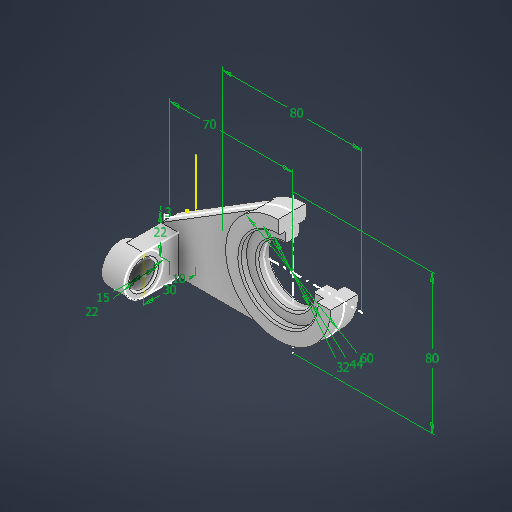
# Autodesk Inventor part: Day02_Task02
Saved by Autodesk Inventor 2026.3 (Build 303398000, 398)
## iProperties
Created: 2026-08-05
Part Number: Day02_Task02
Material: 일반
Document SubType Name: Modeling
Designer: hojin
Density: 1 g/cm^3
Appearance: 기본값
Author: hojin
Autodesk Inventor part; units mm, degrees
ref_plane "YZ Plane" through (0, 0, 0) normal (1, 0, 0) x (0, 1, 0)
ref_plane "XZ Plane" through (0, 0, 0) normal (0, 1, 0) x (-1, 0, 0)
ref_plane "XY Plane" through (0, 0, 0) normal (0, 0, 1) x (1, 0, 0)
sketch "스케치1" plane through (0, 0, 0) normal (0, 1, 0) x (-1, 0, 0)
  point P0 (0, 0)
sketch "스케치2" plane through (0, 0, 0) normal (0, 0, 1) x (1, 0, 0)
  arc A0 (0, 16) -> (16, 0) centre (0, 0) ccw
  arc A1 (0, 22) -> (22, 0) centre (0, 0) ccw
  arc A2 (0, 30) -> (30, 0) centre (0, 0) ccw
  line L0 (-70, -8) -> (-60, -8)
  line L1 (-60, -8) -> (-60, -30)
  line L2 (-60, -30) -> (-70, -30)
  line L3 (-70, -30) -> (-70, -8)
  line L4 (-70, -8) -> (-15.7735, 25.5185)
  line L5 (-70, -30) -> (0, -30)
  line L6 (-73, -8) -> (-70, -8)
  line L7 (-73, -8) -> (-73, -30)
  line L8 (-67, -30) -> (-73, -30)
  line L9 (0, 40) -> (0, -40)
  line L10 (-40, 0) -> (40, 0)
  point P0 (-71.5, -8)
  dimension "d0" = 32
  dimension "d1" = 44
  dimension "d2" = 60
  dimension "d4" = 22
  dimension "d5" = 70
  dimension "d7" = 10
  dimension "d8" = 3
  dimension "d13" = 80
  dimension "d14" = 80
  constraints: 22 end point, 8 point on circle, 6 point on line, 5 coincident, 4 midpoint, 3 centre point, 3 horizontal, 2 parallel, 2 perpendicular, 2 tangent, 2 vertical, 1 collinear
  measures "d0" diameter of A0
  measures "d1" diameter of A1
  measures "d2" diameter of A2
  measures "d4" distance of L0.start L2.end
  measures "d5" horizontal distance of L0.start point (0, 0)
  measures "d7" distance of L1.end L2.end
  measures "d8" distance of L6.start L0.start
  measures "d13" distance of L9.start L9.end
  measures "d14" distance of L10.start L10.end
extrude "돌출3" add sketch "스케치2" along normal mid plane 8 contours A0 L10 A1 L9 | A0 L9 A1 L10 | A0 L10 A1 L9
extrude "돌출4" add sketch "스케치2" along normal mid plane 16 contours A1 L10 A2 L9 | A1 L9 A2 L10 | A1 L10 A2 L9
extrude "돌출5" add sketch "스케치2" along normal mid plane 10 contours A2 L5 L1 L0 L4
extrude "돌출6" add sketch "스케치2" against normal blind 5 contours L0 L1 L2 L3
extrude "돌출7" add sketch "스케치2" along normal blind 25 contours L0 L1 L2 L3
sketch "스케치4" plane through (-60, -30, 5) normal (1, 0, 0) x (0, 0, -1)
  circle A0 centre (-20, 11) radius 11
  circle A1 centre (-20, 11) radius 7.5
  line L0 (-20, 0) -> (-20, 22) projected
  line L1 (10, 0) -> (10, 55.5185) projected
  line L2 (10, 0) -> (-20, 0)
  line L3 (10, 22) -> (-20, 22)
  point P0 (5, 30)
  point P1 (-5, 0)
  point P2 (-20, 18.5)
  point P3 (-20, 3.5)
  dimension "d28" = 22
  dimension "d29" = 15
  dimension "d30" = 30
  constraints: 4 end point, 2 centre point, 2 horizontal, 2 midpoint, 2 tangent, 1 concentric, 1 parallel, 1 point on line
  measures "d28" diameter of A0
  measures "d29" diameter of A1
  measures "d30" distance of L1.start L2.end
extrude "돌출8" add sketch "스케치4" against normal blind 13 contours A0 L0 A1 | L0 A1 A0
extrude "돌출9" cut sketch "스케치4" against normal blind 13 contours A1 L0 picked at (-15.876, 12.5587)
fillet "모깎기1" radius 1 6 edges at (-11.3137, -11.3137, 4) (-15.5563, -15.5563, 8) (-60, -11.5, 25) (-11.3137, -11.3137, -4) (-15.5563, -15.5563, -8) (-73, -19, 32.5)
